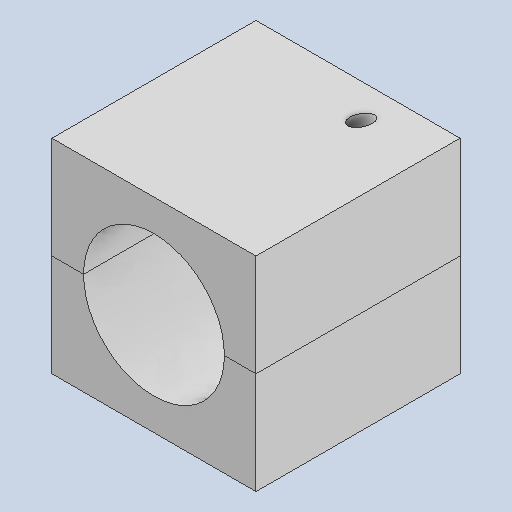
# Autodesk Inventor part: Vŕtnaie
Saved by Autodesk Inventor 2025 (Build 290162000, 162)
## iProperties
Created: 2025-03-25
Part Number: Vŕtnaie
Material: Generic
Document SubType Name: Sheet Metal
Designer: Pravoslav
Density: 1 g/cm^3
Sheet Metal Rule: Default_mm
Appearance: Default
Author: Pravoslav
Autodesk Inventor part; units mm, degrees
ref_plane "YZ Plane" through (0, 0, 0) normal (1, 0, 0) x (0, 1, 0)
ref_plane "XZ Plane" through (0, 0, 0) normal (0, 1, 0) x (-1, 0, 0)
ref_plane "XY Plane" through (0, 0, 0) normal (0, 0, 1) x (1, 0, 0)
sketch "Sketch1" plane through (0, 0, 0) normal (0, 1, 0) x (-1, 0, 0)
  line L0 (15, 15) -> (-15, 15)
  line L1 (-15, 15) -> (-15, -15)
  line L2 (-15, -15) -> (15, -15)
  line L3 (15, -15) -> (15, 15)
  line L4 (15, 15) -> (-15, -15) construction
  line L5 (-15, 15) -> (15, -15) construction
  point P0 (0, 0)
  dimension "d0" = 30
  dimension "d1" = 30
  constraints: 12 end point, 2 midpoint, 2 parallel, 1 horizontal, 1 perpendicular
  measures "d0" distance of L2.end L1.end
  measures "d1" distance of L1.end L0.end
extrude "Extrusion1" add sketch "Sketch1" along normal blind 30
sketch "Sketch2" plane through (-15, 0, 15) normal (0, 0, 1) x (1, 0, 0)
  circle A0 centre (15, 15) radius 10.35
  line L0 (0, 0) -> (30, 0) projected
  line L1 (0, 0) -> (0, 30) projected
  line L2 (15, 15) -> (20.4596, 0)
  line L3 (15, 15) -> (15, 0)
  line L4 (15, 15) -> (15, 30)
  line L5 (30, 30) -> (0, 30) projected
  line L6 (15, 15) -> (20.4596, 30)
  dimension "d4" = 15
  dimension "d5" = 15
  dimension "d6" = 20.7
  dimension "d9" = 20
  dimension "d10" = 20
  dimension "d11" = 15
  dimension "d12" = 15
  constraints: 8 end point, 1 centre point, 1 midpoint
  measures "d4" distance from line of L0 L2.start
  measures "d5" distance from line of L2.start L1
  measures "d6" diameter of A0
  measures "d9" angle of L3 L2
  measures "d10" angle of L4 L6
  measures "d11" vertical distance of L2.start L2.end
  measures "d12" vertical distance of L2.start L6.end
extrude "Extrusion2" cut sketch "Sketch2" against normal through all contours A0 L2 L6 | L6 L4 A0 | A0 L3 L2 | L4 L3 A0
sketch "Sketch3" plane through (0, 0, 0) normal (0, -1, 0) x (1, 0, 0)
  line L0 (-15, 15) -> (15, 15) projected
  line L1 (5.46, 15) -> (5.46, -15)
  line L2 (15, -15) -> (-15, -15) projected
  line L3 (15, 15) -> (15, -15) projected
  point P0 (0, 0)
  dimension "d13" = 9.54
  constraints: 2 end point, 2 point on line, 1 vertical
  measures "d13" distance between parallel lines of L3 L1
sketch "Sketch4" plane through (-15, 0, -15) normal (-1, 0, 0) x (0, 0, 1)
  line L0 (30, 0) -> (0, 0) projected
  line L1 (15, 15) -> (0, 0)
  line L2 (0, 30) -> (30, 30) projected
  line L3 (30, 0) -> (30, 30) projected
  point P0 (15, 0)
  dimension "d14" = 15
  dimension "d15" = 15
  dimension "d16" = 45
  constraints: 2 end point
  measures "d14" distance from line of L2 L1.start
  measures "d15" distance from line of L3 L1.start
  measures "d16" angle of L0 L1
sketch "Sketch5" plane through (0, 0, 0) normal (0, -1, 0) x (1, 0, 0)
  line L0 (15, -15) -> (-15, -15) projected
  line L1 (15, 15) -> (15, -15) projected
  point P0 (0, 0)
  point P1 (5.46, -10)
  dimension "d17" = 5
  dimension "d18" = 9.54
  measures "d17" distance from line of L0 point (5.46, -10)
  measures "d18" distance from line of L1 point (5.46, -10)
hole "Hole1" at (5.46, 0, -10) direction (-0.2419308, 0.6644528, 0.707087) diameter 2.3 depth 30.606
hole "Hole2" at (5.46, 0, -10) direction (0.2419308, -0.6644528, -0.707087) diameter 2.3 end through all
ref_plane "Work Plane1" through (0, 15, 0) normal (0, -1, 0) x (1, 0, 0)
mirror "Mirror1" about plane through (0, 15, 0) normal (0, -1, 0) of "Hole1", "Hole2"
sketch "Sketch8" plane through (-15, 0, 15) normal (0, 0, 1) x (1, 0, 0)
  line L0 (0, 0) -> (0, 30) projected
  line L1 (0, 15) -> (30, 15)
  line L2 (30, 0) -> (30, 30) projected
  line L3 (0, 0) -> (30, 0) projected
  point P0 (15, 0)
  point P1 (15, 0)
  dimension "d55" = 90
  dimension "d56" = 15
  constraints: 3 midpoint, 2 end point
  measures "d55" angle of L1 L0
  measures "d56" distance from line of point (15, 0) L1
split body "Split3" sketch "Sketch8" result two bodies curves L1 first body at (7.1304, 23.178, -1.3765)
equation "\"d43\" = Thickness"
equation "\"BendRadius\" = Thickness"
equation "\"BendReliefWidth\" = Thickness"
equation "\"BendReliefDepth\" = 0.5 * Thickness"
equation "\"CornerReliefSize\" = 4 * Thickness"
equation "\"MinimumRemnant\" = 2 * Thickness"
equation "\"TransitionRadius\" = BendRadius"
equation "\"JacobiRadiusSize\" = BendRadius"
equation "\"GapSize\" = Thickness"
equation "\"Thickness\" = 0.5"
body "Solid6"
body "Solid7"
